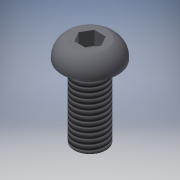
# Autodesk Inventor part: 24-118-8
Saved by Autodesk Inventor 2018 (Build 220105000, 105)
## iProperties
Created: 2004-10-14
Part Number: 24-118-8
Material: Steel, High Strength Low Alloy
Document SubType Name: Modeling
Designer: Autodesk, Inc.
Manufacturer: Standard
Standards Organization: Custom
Description: SCREW, PARKER IPS, BUTTON HEAD, M8X18
Catalog Web Link: http://www.parker.com/ead/cm1.asp?cmid=809
Vendor: PARKER IPS
Mass: 10.8823 g
Surface Area: 9.37524 cm^2
Volume: 1.38805 cm^3
Density: 7.84 g/cm^3
Appearance: Metal (Polished)
CAGE: 1LJX3
Dept. ID: Product Design
Description #2: ---
Finish #1: ---
Finish #2: ---
Material ID: ---
Project Number: ---
Author: Autodesk, Inc.
Autodesk Inventor part; units mm, degrees
ref_plane "YZ Plane" through (0, 0, 0) normal (1, 0, 0) x (0, 1, 0)
ref_plane "XZ Plane" through (0, 0, 0) normal (0, 1, 0) x (-1, 0, 0)
sketch "Sketch1" plane through (0, 0, 0) normal (0, 0, 1) x (1, 0, 0)
  circle A0 centre (0, 0) radius 4
  dimension "Dia" = 8
  constraints: 1 centre point, 1 coincident
  measures "Dia" diameter of A0
extrude "Base" add sketch "Sketch1" against normal blind 18
ref_plane "Hex Key Sketch Plane" through (0, 0, 4.4) normal (0, 0, 1) x (1, 0, 0)
sketch "Sketch2" plane through (0, 0, 0) normal (0, 1, 0) x (-1, 0, 0)
  line L0 (0, -0.969) -> (0, 5.8139) projected
  line L1 (-4, 0) -> (4, 0) projected
  line L2 (0, 0) -> (7, 0)
  line L3 (7, 0) -> (7, 0.44)
  arc A0 (7, 0.44) -> (4.2, 4.4) centre (2.7997, 0.44) ccw
  line L4 (4.2, 4.4) -> (0, 4.4)
  line L5 (0, 4.4) -> (0, 0)
  dimension "d3" = 4.4
  dimension "d4" = 0.44
  dimension "d5" = 14
  dimension "d6" = 2.8
  constraints: 8 end point, 2 collinear, 2 perpendicular, 2 point on circle, 1 centre point, 1 midpoint, 1 point on line, 1 tangent
  measures "d3" distance between parallel lines of L2 L4
  measures "d4" distance of L2.end L3.end
  measures "d5" diameter of L3 L0
  measures "d6" distance from line of L3 L4.start
revolve "Button Head" add sketch "Sketch2" angle 360 about axis through (0, 0, -10) along (0, 0, 1)
sketch "Sketch4" plane through (0, 0, 0) normal (0, 1, 0) x (-1, 0, 0)
  line L0 (0, -0.88) -> (0, 5.28) projected
  line L1 (-4, 0) -> (4, 0) projected
  line L2 (0, 0) -> (7, 0)
  line L3 (7, 0) -> (7, 4.4)
  line L4 (7, 4.4) -> (0, 4.4)
  line L5 (0, 4.4) -> (0, 0)
  dimension "d13" = 4.4
  dimension "d14" = 14
  constraints: 8 end point, 2 parallel, 1 horizontal, 1 midpoint, 1 perpendicular
  measures "d13" distance of L2.end L3.end
  measures "d14" diameter of L3 L0
revolve "Cap Head" [suppressed]
sketch "Sketch3" plane through (0, 0, 0) normal (0, 1, 0) x (-1, 0, 0)
  line L0 (0, -21.6) -> (0, 3.6) projected
  line L1 (-4, 0) -> (4, 0) projected
  line L2 (4, 0) -> (4, -18) projected
  line L3 (0, 0) -> (7, 0)
  line L4 (7, 0) -> (7, -0.44)
  line L5 (7, -0.44) -> (4, -4.4)
  line L6 (4, -4.4) -> (0, -4.4)
  line L7 (0, 0) -> (0, -4.4)
  dimension "d9" = 4.4
  dimension "d10" = 14
  dimension "d11" = 0.44
  constraints: 10 end point, 3 point on line, 2 perpendicular, 1 collinear, 1 midpoint
  measures "d9" distance between parallel lines of L6 L3
  measures "d10" diameter of L4 L0
  measures "d11" distance of L3.end L4.end
revolve "Flat Head" [suppressed]
sketch "Sketch5" plane through (0, 0, 4.4) normal (0, 0, 1) x (1, 0, 0)
  line L0 (1.4434, 2.5) -> (2.8868, 0)
  line L1 (2.8868, 0) -> (1.4434, -2.5)
  line L2 (1.4434, -2.5) -> (-1.4434, -2.5)
  line L3 (-1.4434, -2.5) -> (-2.8868, 0)
  line L4 (-2.8868, 0) -> (-1.4434, 2.5)
  line L5 (-1.4434, 2.5) -> (1.4434, 2.5)
  point P0 (0, 0)
  point P1 (0, 0)
  dimension "d16" = 5
  constraints: 12 end point, 1 coincident, 1 horizontal, 11 other
  measures "d16" distance between parallel lines of L2 L5
extrude "Hex Socket" cut sketch "Sketch5" against normal blind 3.52
thread "Thread1" size "M8x1.25" class "6g" standard "ANSI Metric M Profile" full length
equation "\"d3\" = H_K"
equation "\"d4\" = 0.1 * H_K"
equation "\"d5\" = Dk"
equation "\"d6\" = 0.2 * Dk"
equation "\"d13\" = H_K"
equation "\"d14\" = Dk"
equation "\"d9\" = H_K"
equation "\"d10\" = Dk"
equation "\"d11\" = 0.1 * H_K"
equation "\"d16\" = H_S"
equation "\"d17\" = 0.8 * H_K"
equation "\"Dk\" = 14"
equation "\"H_K\" = 4.4"
equation "\"H_S\" = 5"
equation "\"HexStartHeight\" = H_K"
body "Solid1"
